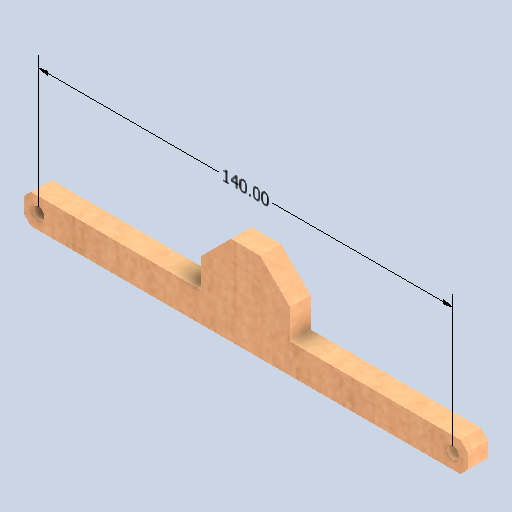
# Autodesk Inventor part: Lever
Saved by Autodesk Inventor 2023.1 (Build 271208000, 208)
## iProperties
Created: 2022-10-28
Part Number: Lever
Material: MDF Medium Density Fiberboard
Document SubType Name: Modeling
Designer: Daniel Peña
Density: 0.8 g/cm^3
Appearance: Cherry - Natural Low Gloss
Author: Daniel Peña
Autodesk Inventor part; units mm, degrees
ref_plane "YZ Plane" through (0, 0, 0) normal (1, 0, 0) x (0, 1, 0)
ref_plane "XZ Plane" through (0, 0, 0) normal (0, 1, 0) x (-1, 0, 0)
ref_plane "XY Plane" through (0, 0, 0) normal (0, 0, 1) x (1, 0, 0)
sketch "Sketch1" plane through (0, 0, 0) normal (0, 0, 1) x (1, 0, 0)
  line L0 (-3.1319, 102.9805) -> (141.8681, 102.9805)
  line L1 (144.3681, 100.4805) -> (144.3681, 95.4805)
  line L2 (141.8681, 92.9805) -> (-3.1319, 92.9805)
  line L3 (-5.6319, 95.4805) -> (-5.6319, 100.4805)
  line L4 (141.8681, 102.9805) -> (144.3681, 100.4805)
  line L5 (-3.1319, 102.9805) -> (-5.6319, 100.4805)
  line L6 (-5.6319, 95.4805) -> (-3.1319, 92.9805)
  line L7 (141.8681, 92.9805) -> (144.3681, 95.4805)
  line L8 (69.3681, 92.9805) -> (69.3681, 132.9805) construction
  line L9 (84.3681, 102.9805) -> (54.3681, 102.9805)
  line L10 (54.3681, 102.9805) -> (54.3681, 112.9805)
  line L11 (64.3681, 122.9805) -> (74.3681, 122.9805)
  line L12 (84.3681, 112.9805) -> (84.3681, 102.9805)
  line L13 (74.3681, 122.9805) -> (84.3681, 112.9805)
  line L14 (54.3681, 112.9805) -> (64.3681, 122.9805)
  circle A0 centre (69.3681, 107.9805) radius 12.5 construction
  point P0 (0, 0)
  point P1 (-5.6319, 102.9805)
  point P2 (144.3681, 92.9805)
  point P3 (144.3681, 102.9805)
  point P4 (-5.6319, 92.9805)
  point P5 (54.3681, 122.9805)
  point P6 (84.3681, 122.9805)
  dimension "d0" = 150
  dimension "d1" = 10
  dimension "d2" = 2.5
  dimension "d3" = 2.5
  dimension "d4" = 2.5
  dimension "d5" = 2.5
  dimension "d6" = 2.5
  dimension "d7" = 2.5
  dimension "d8" = 2.5
  dimension "d9" = 2.5
  dimension "d12" = 40
  dimension "d13" = 30
  dimension "d14" = 20
  dimension "d15" = 15
  dimension "d16" = 10
  dimension "d17" = 10
  dimension "d18" = 10
  dimension "d19" = 10
  dimension "d20" = 25
  constraints: 30 end point, 14 point on line, 4 parallel, 2 horizontal, 2 perpendicular, 1 centre point, 1 midpoint, 1 vertical
  measures "d0" distance of point (144.368, 92.98) point (-5.632, 92.98)
  measures "d1" distance of point (144.368, 102.98) point (144.368, 92.98)
  measures "d2" distance of L0.end point (144.368, 102.98)
  measures "d3" distance of L1.start point (144.368, 102.98)
  measures "d4" distance of L0.start point (-5.632, 102.98)
  measures "d5" distance of L3.end point (-5.632, 102.98)
  measures "d6" distance of L3.start point (-5.632, 92.98)
  measures "d7" distance of L2.end point (-5.632, 92.98)
  measures "d8" distance of L2.start point (144.368, 92.98)
  measures "d9" distance of L1.end point (144.368, 92.98)
  measures "d12" distance of L8.start L8.end
  measures "d13" distance of point (54.368, 122.98) point (84.368, 122.98)
  measures "d14" distance of L9.end point (54.368, 122.98)
  measures "d15" distance between parallel lines of L10 L8
  measures "d16" distance of L11.end point (84.368, 122.98)
  measures "d17" distance of L12.start point (84.368, 122.98)
  measures "d18" distance of L10.end point (54.368, 122.98)
  measures "d19" distance of L11.start point (54.368, 122.98)
  measures "d20" diameter of A0
extrude "Extrusion1" add sketch "Sketch1" along normal blind 7
sketch "Sketch2" plane through (0, 0, 7) normal (0, 0, 1) x (1, 0, 0)
  line L0 (74.3681, 122.9805) -> (64.3681, 122.9805) construction
  line L1 (69.3681, 122.9805) -> (69.3681, 92.9805) construction
  line L2 (-3.1319, 92.9805) -> (141.8681, 92.9805) construction
  line L3 (-5.6319, 100.4805) -> (-5.6319, 95.4805) construction
  point P0 (0, 0)
  point P1 (-0.6319, 97.9805)
  point P2 (139.3681, 97.9805)
  dimension "d21" = 5
  constraints: 2 end point, 2 midpoint, 1 symmetric about line
  measures "d21" distance from line of L3 point (-0.632, 97.98)
hole "Hole1" at (-0.6319, 97.9805, 7) at (139.3681, 97.9805, 7) direction (0, 0, -1) diameter 4 end through all
equation "\"d2\" = d4"
equation "\"d3\" = d2"
equation "\"d5\" = d4"
equation "\"d6\" = d4"
equation "\"d7\" = d6"
equation "\"d8\" = d4"
equation "\"d9\" = d8"
equation "\"d17\" = d16"
equation "\"d18\" = d16"
equation "\"d19\" = d18"
body "Solid1"
